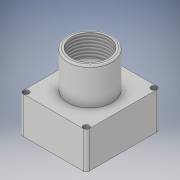
# Autodesk Inventor part: Práctica 1 - Melany Escobar
Saved by Autodesk Inventor 2019.1 (Build 231200000, 200)
## iProperties
Created: 2024-02-03
Part Number: Práctica 1 - Melany Escobar
Material: Generic
Document SubType Name: Modeling
Designer: clariheelen
Density: 1 g/cm^3
Appearance: Default
Author: clariheelen
Autodesk Inventor part; units mm, degrees
ref_plane "YZ Plane" through (0, 0, 0) normal (1, 0, 0) x (0, 1, 0)
ref_plane "XZ Plane" through (0, 0, 0) normal (0, 1, 0) x (-1, 0, 0)
ref_plane "XY Plane" through (0, 0, 0) normal (0, 0, 1) x (1, 0, 0)
sketch "Sketch2" plane through (0, 0, 0) normal (0, 1, 0) x (-1, 0, 0)
  line L0 (45, 50) -> (-45, 50)
  line L1 (-45, 50) -> (-45, -50)
  line L2 (-45, -50) -> (45, -50)
  line L3 (45, -50) -> (45, 50)
  line L4 (45, 50) -> (-45, -50) construction
  line L5 (-45, 50) -> (45, -50) construction
  point P0 (0, 0)
  dimension "d0" = 90
  dimension "d1" = 100
  constraints: 12 end point, 2 midpoint, 2 parallel, 1 horizontal, 1 perpendicular
  measures "d0" distance of L2.end L1.end
  measures "d1" distance of L1.end L0.end
extrude "Extrusion1" add sketch "Sketch2" along normal blind 50
sketch "Sketch4" plane through (0, 50, 0) normal (0, 1, 0) x (1, 0, 0)
  point P0 (0, 0)
  point P1 (40.9905, 45.9844)
hole "Hole1" at (40.9905, 50, -45.9844) direction (0, -1, 0) diameter 8 end through all
sketch "Sketch5" plane through (0, 0, 0) normal (0, -1, 0) x (1, 0, 0)
  point P0 (0, 0)
  point P1 (-40.9769, 45.9697)
hole "Hole2" at (-40.9769, 0, 45.9697) direction (0, 1, 0) diameter 8 end through all
sketch "Sketch6" plane through (0, 0, 0) normal (0, -1, 0) x (1, 0, 0)
  point P0 (0, 0)
  point P1 (-40.9656, -45.9539)
hole "Hole3" at (-40.9656, 0, -45.9539) direction (0, 1, 0) diameter 8 end through all
sketch "Sketch7" plane through (0, 50, 0) normal (0, 1, 0) x (1, 0, 0)
  point P0 (0, 0)
  point P1 (40.9483, -45.9561)
hole "Hole4" at (40.9483, 50, 45.9561) direction (0, -1, 0) diameter 8 end through all
thread "Thread1" size "M8x1.25" class "6H" standard "ANSI Metric M Profile" full length
thread "Thread2" size "M8x1.25" class "6H" standard "ANSI Metric M Profile" full length
thread "Thread3" size "M8x1.25" class "6H" standard "ANSI Metric M Profile" full length
thread "Thread4" size "M8x1.25" class "6H" standard "ANSI Metric M Profile" full length
fillet "Fillet1" radius 4 1 edges at (45, 25, -50)
fillet "Fillet2" radius 4 1 edges at (-45, 25, -50)
fillet "Fillet3" radius 4 1 edges at (-45, 25, 50)
fillet "Fillet4" radius 4 1 edges at (45, 25, 50)
sketch "Sketch9" plane through (0, 50, 0) normal (0, 1, 0) x (1, 0, 0)
  circle A0 centre (0, 0) radius 30
  dimension "d44" = 60
  constraints: 1 centre point, 1 coincident
  measures "d44" diameter of A0
extrude "Extrusion2" add sketch "Sketch9" along normal blind 50
sketch "Sketch10" plane through (0, 100, 0) normal (0, 1, 0) x (1, 0, 0)
  circle A0 centre (0, 0) radius 25
  dimension "d47" = 50
  constraints: 1 centre point, 1 coincident
  measures "d47" diameter of A0
extrude "Extrusion3" cut sketch "Sketch10" against normal blind 30
thread "Thread5" size "M50x4" class "6H" standard "ANSI Metric M Profile" full length
fillet "Fillet5" radius 2.5 1 edges at (-30, 100, 0)
body "Solid1"
